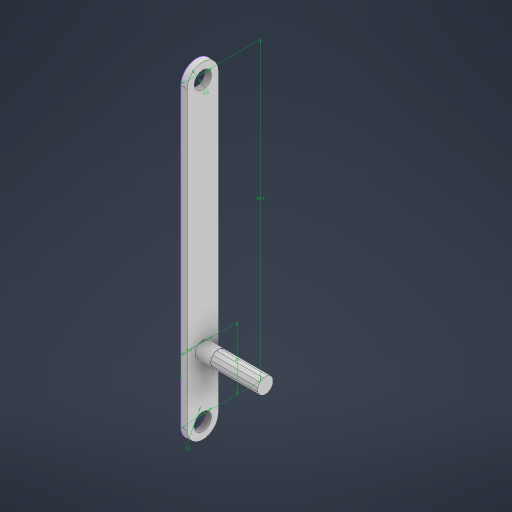
# Autodesk Inventor part: gunholder_v3 L
Saved by Autodesk Inventor 2024.1 (Build 281209000, 209)
## iProperties
Created: 2023-07-11
Part Number: gunholder_v3 L
Material: 일반
Document SubType Name: Modeling
Designer: 6gioc
Density: 1 g/cm^3
Appearance: 기본값
Author: 6gioc
## iProperties of the stored document gunholder_v3 L_3D 인쇄.ipt
Created: 2023-09-27
Part Number: gunholder_v3 L_3D 인쇄
Material: 일반
Document SubType Name: Modeling
Designer: 6gioc
Density: 1 g/cm^3
Appearance: 기본값
Author: 6gioc
Autodesk Inventor part; units mm, degrees
ref_plane "YZ Plane" through (0, 0, 0) normal (1, 0, 0) x (0, 1, 0)
ref_plane "XZ Plane" through (0, 0, 0) normal (0, 1, 0) x (-1, 0, 0)
ref_plane "XY Plane" through (0, 0, 0) normal (0, 0, 1) x (1, 0, 0)
sketch "스케치1" plane through (0, 0, 0) normal (1, 0, 0) x (0, 1, 0)
  circle A0 centre (0, 0) radius 2.5
  line L0 (2.4148, 0.647) -> (2.4148, -0.647)
  line L1 (2.4148, -0.647) -> (1.7678, -1.7678)
  line L2 (1.7678, -1.7678) -> (0.647, -2.4148)
  line L3 (0.647, -2.4148) -> (-0.647, -2.4148)
  line L4 (-0.647, -2.4148) -> (-1.7678, -1.7678)
  line L5 (-1.7678, -1.7678) -> (-2.4148, -0.647)
  line L6 (-2.4148, -0.647) -> (-2.4148, 0.647)
  line L7 (-2.4148, 0.647) -> (-1.7678, 1.7678)
  line L8 (-1.7678, 1.7678) -> (-0.647, 2.4148)
  line L9 (-0.647, 2.4148) -> (0.647, 2.4148)
  line L10 (0.647, 2.4148) -> (1.7678, 1.7678)
  line L11 (1.7678, 1.7678) -> (2.4148, 0.647)
  circle A1 centre (0, 0) radius 5
  circle A2 centre (-20, 0) radius 5
  circle A3 centre (74.5, 0) radius 5
  circle A4 centre (74.5, 0) radius 2.75
  circle A5 centre (-20, 0) radius 2.75
  line L12 (74.5, 5) -> (-20, 5)
  line L13 (-20, -5) -> (74.5, -5)
  point P0 (2.5, 0)
  dimension "d0" = 5
  dimension "d1" = 10
  dimension "d2" = 10
  dimension "d3" = 20
  dimension "d4" = 10
  dimension "d5" = 94.5
  dimension "d6" = 5.5
  dimension "d7" = 5.5
  constraints: 28 end point, 6 centre point, 6 coincident, 6 point on circle, 2 tangent, 1 horizontal, 25 other
  measures "d0" diameter of A0
  measures "d1" diameter of A1
  measures "d2" diameter of A2
  measures "d3" distance of A2.centre A1.centre
  measures "d4" diameter of A3
  measures "d5" distance of A2.centre A3.centre
  measures "d6" diameter of A4
  measures "d7" diameter of A5
extrude "돌출1" add sketch "스케치1" along normal blind 2 contours A0 L0 | L11 A0 | A0 L1 | L10 A0 | A0 L2 | L9 A0 | A0 L3 | L8 A0 | A0 L4 | L7 A0 | A0 L5 | L6 A0 | A1 | A1 L12 A3 L13 | A1 L13 A2 L12 | A3 | A2
extrude "돌출2" add sketch "스케치1" along normal blind 7 contours A0 L0 | L11 A0 | L0 L1 L2 L3 L4 L5 L6 L7 L8 L9 L10 L11 | A0 L1 | L10 A0 | A0 L2 | L9 A0 | A0 L3 | L8 A0 | A0 L4 | L7 A0 | A0 L5 | L6 A0
extrude "돌출3" add sketch "스케치1" along normal blind 22 contours L0 L1 L2 L3 L4 L5 L6 L7 L8 L9 L10 L11
equation "\"clearance\" = 1"
